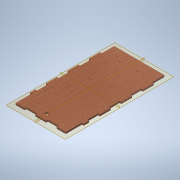
# Autodesk Inventor part: Plaat boven
Saved by Autodesk Inventor 2021 (Build 250183000, 183)
## iProperties
Manager: PJ / DCS
Company: Emmaüs Bovenbouw Aalter
Created: 2021-01-09
Part Number: Plaat boven
Material: S235
Catalog Web Link: http://emmausbovenbouw.op-weg.be/
Vendor: Emmaüsinstituut Bovenbouw Aalter
Document SubType Name: Modeling
Designer: Antho
Engineer: Declercq St.
Manufacturer: Standard
Standards Organization: Custom
Density: 7.86 g/cm^3
Appearance: White Oak - Natural Medium Gloss
Title: Algemene titel
Subject: Specifieke titel
Author: Antho
Keywords: Ruwe Ø xxxxx
Comments: Opmerking
Autodesk Inventor part; units mm, degrees
sketch "Sketch1" plane through (0, 0, 0) normal (0, 0, 1) x (1, 0, 0)
  line L0 (0, 2.8582) -> (0, -2.8582) construction
  line L1 (-5.7775, 0) -> (5.7775, 0) construction
  line L2 (-75, -137.5) -> (75, -137.5)
  line L3 (75, -137.5) -> (75, 137.5)
  line L4 (75, 137.5) -> (-75, 137.5)
  line L5 (-75, 137.5) -> (-75, -137.5)
  line L6 (-75, -137.5) -> (75, 137.5) construction
  line L7 (75, -137.5) -> (-75, 137.5) construction
  point P0 (0, 0)
  point P1 (0, 0)
  dimension "d0" = 150
  dimension "d1" = 275
  constraints: 16 end point, 4 midpoint, 2 horizontal, 2 parallel, 1 coincident, 1 perpendicular, 1 vertical
  measures "d0" distance of L4.end L3.end
  measures "d1" distance of L3.end L2.end
extrude "Extrusion1" add sketch "Sketch1" along normal blind 5
sketch "Sketch2" plane through (0, 0, 5) normal (0, 0, 1) x (1, 0, 0)
  line L0 (0, 0) -> (0, -120)
  circle A0 centre (0, -120) radius 5
  line L1 (-75, 137.5) -> (-75, -137.5) projected
  line L2 (-75, -137.5) -> (-70, -137.5)
  line L3 (-70, -137.5) -> (-70, -92.5)
  line L4 (-70, -92.5) -> (-75, -92.5)
  line L5 (-75, -92.5) -> (-75, -137.5)
  line L6 (-75, -92.5) -> (-75, -77.5)
  line L7 (-75, -77.5) -> (-75, -47.5)
  line L8 (-75, -47.5) -> (-75, -17.5)
  line L9 (-75, -17.5) -> (-75, 12.5)
  line L10 (-75, 12.5) -> (-75, 42.5)
  line L11 (-75, 42.5) -> (-75, 72.5)
  line L12 (-75, 72.5) -> (-75, 102.5)
  line L13 (-75, 102.5) -> (-75, 132.5)
  line L14 (-75, -77.5) -> (-70, -77.5)
  line L15 (-70, -77.5) -> (-70, -47.5)
  line L16 (-70, -47.5) -> (-75, -47.5)
  line L17 (-75, -47.5) -> (-75, -77.5)
  line L18 (-75, -17.5) -> (-70, -17.5)
  line L19 (-70, -17.5) -> (-70, 12.5)
  line L20 (-70, 12.5) -> (-75, 12.5)
  line L21 (-75, 12.5) -> (-75, -17.5)
  line L22 (-75, 42.5) -> (-70, 42.5)
  line L23 (-70, 42.5) -> (-70, 72.5)
  line L24 (-70, 72.5) -> (-75, 72.5)
  line L25 (-75, 72.5) -> (-75, 42.5)
  line L26 (75, 137.5) -> (-75, 137.5) projected
  line L27 (-75, 102.5) -> (-70, 102.5)
  line L28 (-70, 102.5) -> (-70, 137.5)
  line L29 (-70, 137.5) -> (-75, 137.5)
  line L30 (-75, 137.5) -> (-75, 102.5)
  line L31 (75, -137.5) -> (75, 137.5) projected
  line L32 (75, -137.5) -> (75, -92.5)
  line L33 (75, -92.5) -> (75, -77.5)
  line L34 (75, -77.5) -> (75, -47.5)
  line L35 (75, -47.5) -> (75, -17.5)
  line L36 (75, -17.5) -> (75, 12.5)
  line L37 (75, 12.5) -> (75, 42.5)
  line L38 (75, 42.5) -> (75, 72.5)
  line L39 (75, 72.5) -> (75, 102.5)
  line L40 (75, 102.5) -> (75, 132.5)
  line L41 (-75, -137.5) -> (75, -137.5) projected
  line L42 (75, -137.5) -> (70, -137.5)
  line L43 (70, -137.5) -> (70, -92.5)
  line L44 (70, -92.5) -> (75, -92.5)
  line L45 (75, -92.5) -> (75, -137.5)
  line L46 (75, -77.5) -> (70, -77.5)
  line L47 (70, -77.5) -> (70, -47.5)
  line L48 (70, -47.5) -> (75, -47.5)
  line L49 (75, -47.5) -> (75, -77.5)
  line L50 (75, -17.5) -> (70, -17.5)
  line L51 (70, -17.5) -> (70, 12.5)
  line L52 (70, 12.5) -> (75, 12.5)
  line L53 (75, 12.5) -> (75, -17.5)
  line L54 (75, 42.5) -> (70, 42.5)
  line L55 (70, 42.5) -> (70, 72.5)
  line L56 (70, 72.5) -> (75, 72.5)
  line L57 (75, 72.5) -> (75, 42.5)
  line L58 (75, 102.5) -> (70, 102.5)
  line L59 (70, 102.5) -> (70, 137.5)
  line L60 (70, 137.5) -> (75, 137.5)
  line L61 (75, 137.5) -> (75, 102.5)
  line L62 (0, -137.5) -> (-15, -137.5)
  line L63 (-15, -137.5) -> (15, -137.5)
  line L64 (-15, -137.5) -> (-45, -137.5)
  line L65 (-45, -137.5) -> (-45, -132.5)
  line L66 (-45, -132.5) -> (-15, -132.5)
  line L67 (-15, -132.5) -> (-15, -137.5)
  line L68 (15, -137.5) -> (45, -137.5)
  line L69 (45, -137.5) -> (45, -132.5)
  line L70 (45, -132.5) -> (15, -132.5)
  line L71 (15, -132.5) -> (15, -137.5)
  point P0 (-75, -92.5)
  dimension "d4" = 120
  dimension "d5" = 10
  dimension "d6" = 5
  dimension "d7" = 45
  dimension "d9" = 30
  dimension "d10" = 30
  dimension "d11" = 30
  dimension "d12" = 30
  dimension "d13" = 30
  dimension "d14" = 30
  dimension "d15" = 30
  dimension "d16" = 5
  dimension "d17" = 30
  dimension "d18" = 5
  dimension "d19" = 5
  dimension "d20" = 5
  dimension "d21" = 45
  dimension "d23" = 30
  dimension "d24" = 30
  dimension "d25" = 30
  dimension "d26" = 30
  dimension "d27" = 30
  dimension "d28" = 30
  dimension "d29" = 30
  dimension "d30" = 5
  dimension "d31" = 5
  dimension "d32" = 15
  dimension "d33" = 30
  dimension "d34" = 30
  dimension "d35" = 5
  dimension "d36" = 30
  dimension "d37" = 5
  dimension "d40" = 45
  constraints: 136 end point, 24 parallel, 12 horizontal, 12 perpendicular, 7 point on line, 1 centre point, 1 coincident, 1 midpoint, 1 vertical, 19 other
  measures "d4" distance of L0.start L0.end
  measures "d5" diameter of A0
  measures "d6" distance of L4.end L3.end
  measures "d7" distance of L3.end L2.end
  measures "d9" distance of L6.end L7.end
  measures "d10" distance of L7.end L8.end
  measures "d11" distance of L8.end L9.end
  measures "d12" distance of L9.end L10.end
  measures "d13" distance of L10.end L11.end
  measures "d14" distance of L11.end L12.end
  measures "d15" distance of L12.end L13.end
  measures "d16" distance of L16.end L15.end
  measures "d17" distance of L15.end L14.end
  measures "d18" distance of L20.end L19.end
  measures "d19" distance of L24.end L23.end
  measures "d20" distance of L29.end L28.end
  measures "d21" distance of L32.start L32.end
  measures "d23" distance of L33.end L34.end
  measures "d24" distance of L34.end L35.end
  measures "d25" distance of L35.end L36.end
  measures "d26" distance of L36.end L37.end
  measures "d27" distance of L37.end L38.end
  measures "d28" distance of L38.end L39.end
  measures "d29" distance of L39.end L40.end
  measures "d30" distance of L43.end L44.end
  measures "d31" distance of L47.end L48.end
  measures "d32" distance of L62.start L62.end
  measures "d33" distance of L62.end L63.end
  measures "d34" distance of L65.end L66.end
  measures "d35" distance of L64.end L65.end
  measures "d36" distance of L70.end L69.end
  measures "d37" distance of L69.end L68.end
  measures "d40" distance of L42.end L43.end
extrude "Extrusion2" cut sketch "Sketch2" against normal blind 8 contours A0 | L26 L28 L27 L1 | L26 L31 L58 L59 | L24 L23 L22 L1 | L20 L19 L18 L1 | L31 L54 L55 L56 | L16 L15 L14 L1 | L31 L50 L51 L52 | L4 L3 L2 L1 | L31 L46 L47 L48 | L31 L41 L43 L44 | L65 L66 L67 L41 | L41 L71 L70 L69
sketch "Sketch3" plane through (0, 0, 5) normal (0, 0, 1) x (1, 0, 0)
  line L0 (70, 137.5) -> (-70, 137.5) projected
  line L1 (0, 137.5) -> (0, 107.5)
  line L2 (0, 107.5) -> (-24.14, 107.5)
  line L3 (0, 107.5) -> (24.14, 107.5)
  line L4 (24.14, 107.5) -> (24.14, 32.57)
  line L5 (-24.14, 107.5) -> (-24.14, 24.95)
  point P0 (0, 0)
  dimension "d42" = 30
  dimension "d43" = 24.14
  dimension "d44" = 24.14
  dimension "d45" = 74.93
  dimension "d46" = 82.55
  constraints: 10 end point, 4 coincident, 3 vertical, 2 horizontal, 1 midpoint
  measures "d42" distance of L1.start L1.end
  measures "d43" distance of L1.end L2.end
  measures "d44" distance of L1.end L3.end
  measures "d45" distance of L3.end L4.end
  measures "d46" distance of L2.end L5.end
hole "Hole1" at (-24.14, 24.95, 5) at (24.14, 32.57, 5) at (24.14, 107.5, 5) at (-24.14, 107.5, 5) direction (0, 0, -1) diameter 3.27 end through all
body "Solid1"
